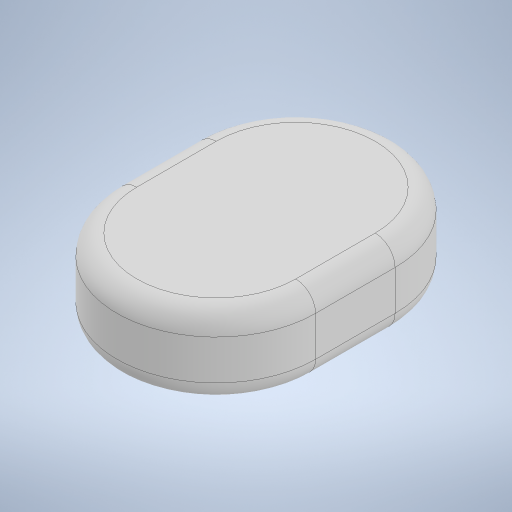
# Autodesk Inventor part: Ползунок
Saved by Autodesk Inventor 2023.1 (Build 271208000, 208)
## iProperties
Created: 2023-07-03
Part Number: Ползунок
Material: Generic
Document SubType Name: Modeling
Designer: adamn
Density: 1 g/cm^3
Appearance: Default
Author: adamn
Autodesk Inventor part; units mm, degrees
ref_plane "YZ Plane" through (0, 0, 0) normal (1, 0, 0) x (0, 1, 0)
ref_plane "XZ Plane" through (0, 0, 0) normal (0, 1, 0) x (-1, 0, 0)
ref_plane "XY Plane" through (0, 0, 0) normal (0, 0, 1) x (1, 0, 0)
sketch "Sketch1" plane through (0, 0, 0) normal (0, 1, 0) x (-1, 0, 0)
  line L0 (0, 0) -> (0, -2) construction
  line L1 (-2.5, 0) -> (-2.5, -2)
  line L2 (2.5, -2) -> (2.5, 0)
  arc A0 (2.5, 0) -> (-2.5, 0) centre (0, 0) ccw
  arc A1 (-2.5, -2) -> (2.5, -2) centre (0, -2) ccw
  point P0 (0, -1)
  dimension "d0" = 2.5
  dimension "d1" = 2
  constraints: 8 end point, 4 point on circle, 4 tangent, 2 centre point, 1 midpoint, 1 parallel, 1 vertical
  measures "d0" radius of A0
  measures "d1" distance of L0.end L0.start
extrude "Extrusion1" add sketch "Sketch1" along normal blind 2
sketch "Sketch2" plane through (0, 2, 0) normal (0, 1, 0) x (1, 0, 0)
  circle A0 centre (0, 1) radius 1.5
  line L0 (-2.5, 2) -> (-2.5, 0) projected
  point P0 (0, 0)
  point P1 (-2.5, 1)
  dimension "d4" = 3
  constraints: 1 centre point, 1 horizontal alignment, 1 midpoint, 1 vertical alignment
  measures "d4" diameter of A0
extrude "Extrusion2" cut sketch "Sketch2" against normal blind 12.25
fillet "Fillet1" radius 0.5 8 edges at (2.5, 2, -1) (0, 2, -4.5) (-2.5, 2, -1) (0, 2, 2.5) (2.5, 0, -1) (0, 0, -4.5) (-2.5, 0, -1) (0, 0, 2.5)
sketch "Sketch3" plane through (0, 2, 0) normal (0, 1, 0) x (1, 0, 0)
  circle A0 centre (0, 1) radius 1.5 projected
  point P0 (0, 0)
extrude "Extrusion3" add sketch "Sketch3" against normal blind 1.5
body "Solid1"
